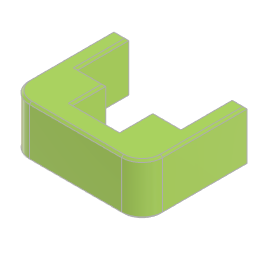
rail_installation_guide_center_x2 (Autodesk Fusion 360 design; units mm, degrees)
Autodesk Fusion 360 part; units mm, degrees
sketch "Sketch1" plane through (0, 0, 0) normal (0, 0, 1) x (1, 0, 0) in component "rail_installation_guide_center_x2"
  line L0 (0, -6.2924) -> (-4.6, -6.2924)
  line L1 (-4.6, -6.2924) -> (-4.6, 0.2076)
  line L2 (-4.6, 0.2076) -> (-10.1, 0.2076)
  line L3 (-10.1, 0.2076) -> (-10.1, 10.2076)
  line L4 (-10.1, 10.2076) -> (-13, 10.2076)
  line L5 (-13, 10.2076) -> (-13, -10.2924)
  line L6 (-13, -10.2924) -> (0, -10.2924)
  line L7 (0, -13) -> (0, 13) construction
  line L8 (0, -6.2924) -> (4.6, -6.2924)
  line L9 (4.6, -6.2924) -> (4.6, 0.2076)
  line L10 (4.6, 0.2076) -> (10.1, 0.2076)
  line L11 (10.1, 0.2076) -> (10.1, 10.2076)
  line L12 (10.1, 10.2076) -> (13, 10.2076)
  line L13 (13, 10.2076) -> (13, -10.2924)
  line L14 (13, -10.2924) -> (0, -10.2924)
  dimension "d9" = 4.6
  dimension "d10" = 6.5
  dimension "d11" = 10
  dimension "d13" = 2.9
  dimension "d14" = 4
  dimension "d15" = 10.1
  constraint horizontal L0
  constraint perpendicular L0 L1
  constraint perpendicular L1 L2
  constraint perpendicular L2 L3
  constraint perpendicular L1 L4
  constraint perpendicular L4 L5
  constraint perpendicular L5 L6
  constraint vertical L7
  constraint symmetric L0.start L7 L8.start
  constraint symmetric L0.end L7 L8.end
  constraint symmetric L1.end L7 L9.end
  constraint symmetric L2.end L7 L10.end
  constraint symmetric L3.end L7 L11.end
  constraint symmetric L4.end L7 L12.end
  constraint symmetric L5.end L7 L13.end
  constraint symmetric L6.end L7 L14.end
  constraint coincident L0.start L7
  constraint coincident L6.end L7
  measures "d9" distance of L0.start L0.end
  measures "d10" distance of L0.end L1.end
  measures "d11" distance of L2.end L3.end
  measures "d13" distance of L3.end L4.end
  measures "d14" distance of L0 L6
  measures "d15" distance of origin L3
extrude "Extrude1" add sketch "Sketch1" along normal mid plane 10 in component "rail_installation_guide_center_x2"
fillet "Fillet1" radius 4 2 edges at (-13, -10.2924, 0) (13, -10.2924, 0) in component "rail_installation_guide_center_x2"
chamfer "Chamfer1" distance 0.4 angle 45 28 edges at (-13, 1.9576, 5) (-11.8284, -9.1208, 5) (0, -10.2924, 5) (11.8284, -9.1208, 5) (13, 1.9576, 5) (-11.55, 10.2076, 5) (-10.1, 5.2076, 5) (-7.35, 0.2076, 5) (-4.6, -3.0424, 5) (0, -6.2924, 5) (4.6, -3.0424, 5) (7.35, 0.2076, 5) (10.1, 5.2076, 5) (11.55, 10.2076, 5) (11.55, 10.2076, -5) (13, 1.9576, -5) (11.8284, -9.1208, -5) (0, -10.2924, -5) (-11.8284, -9.1208, -5) (-13, 1.9576, -5) (-11.55, 10.2076, -5) (-10.1, 5.2076, -5) (-7.35, 0.2076, -5) (-4.6, -3.0424, -5) (0, -6.2924, -5) (4.6, -3.0424, -5) (7.35, 0.2076, -5) (10.1, 5.2076, -5) in component "rail_installation_guide_center_x2"
component "rail_installation_guide_center_x2" placed x (1, 0, 0) y (0, 1, 0) z (0, 0, 1) at (0, 0, 0)
equation "rail_width = 9.0 mm"
equation "tolerance = 0.2 mm"
equation "extrusion_width = 20.00 mm"
equation "arm_length = 10 mm"
equation "rail_depth = 6.5 mm"
equation "tool_thickness = 4 mm"
equation "corner_fillet = 4 mm"
equation "chamfer = 0.4 mm"
equation "d9 = ( rail_width + tolerance ) / 2"
equation "d10 = rail_depth"
equation "d11 = arm_length"
equation "arm_width = 2.9 mm"
equation "d13 = arm_width"
equation "d14 = tool_thickness"
equation "d15 = ( extrusion_width + tolerance ) / 2"
equation "d16 = tool_width / 2"
equation "tool_width = 10 mm"
equation "d20 = corner_fillet"
equation "d21 = chamfer"
